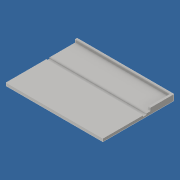
# Autodesk Inventor part: Fixture Base
Saved by Autodesk Inventor 2016 (Build 200138000, 138)
## iProperties
Created: 2016-04-07
Part Number: Fixture Base
Material: Generic
Document SubType Name: Modeling
Designer: Sam Clay
Density: 1 g/cm^3
Appearance: Default
Author: Sam Clay
Autodesk Inventor part; units mm, degrees
ref_plane "YZ Plane" through (0, 0, 0) normal (1, 0, 0) x (0, 1, 0)
ref_plane "XZ Plane" through (0, 0, 0) normal (0, 1, 0) x (-1, 0, 0)
ref_plane "XY Plane" through (0, 0, 0) normal (0, 0, 1) x (1, 0, 0)
sketch "Sketch1" plane through (0, 0, 0) normal (0, 1, 0) x (-1, 0, 0)
  line L0 (0, 0) -> (622.3, 0)
  line L1 (622.3, 0) -> (622.3, 457.2)
  line L2 (622.3, 457.2) -> (0, 457.2)
  line L3 (0, 457.2) -> (0, 0)
  dimension "d0" = 622.3
  dimension "d1" = 457.2
  constraints: 8 end point, 2 parallel, 1 horizontal, 1 perpendicular
  measures "d0" distance of L2.end L1.end
  measures "d1" distance of L1.end L0.end
extrude "Extrusion1" add sketch "Sketch1" along normal blind 19.05
sketch "Sketch2" plane through (0, 19.05, 0) normal (0, 1, 0) x (1, 0, 0)
  line L0 (0, 0) -> (-622.3, 0) projected
  line L1 (-622.3, 0) -> (-622.3, -457.2) projected
  line L2 (0, 0) -> (-622.3, 0)
  line L3 (-622.3, 0) -> (-622.3, -12.7)
  line L4 (-622.3, -12.7) -> (0, -12.7)
  line L5 (0, -12.7) -> (0, 0)
  line L6 (0, 0) -> (-12.7, 0)
  line L7 (-12.7, 0) -> (-12.7, -152.4)
  line L8 (-12.7, -152.4) -> (0, -152.4)
  line L9 (0, -152.4) -> (0, 0)
  circle A0 centre (-15.0509, -15.0058) radius 3.81
  line L10 (-18.0839, -12.7) -> (-12.7, -18.0041) construction
  point P0 (-12.7, -12.7)
  dimension "d4" = 12.7
  dimension "d5" = 12.7
  dimension "d6" = 152.4
  dimension "d74" = 7.62
  constraints: 18 end point, 5 point on line, 4 parallel, 2 horizontal, 2 perpendicular, 2 point on circle, 1 centre point
  measures "d4" distance of L3.end L2.end
  measures "d5" distance of L8.end L7.end
  measures "d6" distance of L7.end L6.end
  measures "d74" diameter of A0
extrude "Extrusion2" add sketch "Sketch2" along normal blind 19.05 contours L5 L4 A0 L7 L0 | L7 A0 L4 L1 L0 | L9 L8 L7 A0 L4 | A0 L4 L7 | L7 L4 A0 | A0 L7 L4 picked at (-12.6177, -12.3088) picked at (-16.0908, -12.4926) picked at (-12.4956, -16.0346)
extrude "Extrusion9" cut sketch "Sketch2" along normal up to next contours A0 L4 L7 | L7 L4 A0 | A0 L7 L4 | L7 A0 L4
sketch "Sketch3" plane through (0, 19.05, 0) normal (0, 1, 0) x (1, 0, 0)
  line L0 (0, -152.4) -> (0, 0) projected
  line L1 (-622.3, -12.7) -> (-622.3, -457.2) projected
  line L2 (0, -197.485) -> (-622.3, -197.485)
  line L3 (-622.3, -197.485) -> (-622.3, -177.8)
  line L4 (-622.3, -177.8) -> (0, -177.8)
  line L5 (0, -177.8) -> (0, -197.485)
  line L6 (0, 0) -> (-622.3, 0) projected
  dimension "d34" = 19.685
  dimension "d66" = 177.8
  constraints: 8 end point, 2 parallel, 2 point on line, 1 horizontal, 1 perpendicular
  measures "d34" distance of L2.end L3.end
  measures "d66" distance between parallel lines of L6 L4
extrude "Extrusion3" cut sketch "Sketch3" against normal blind 7.62
body "Solid1"
